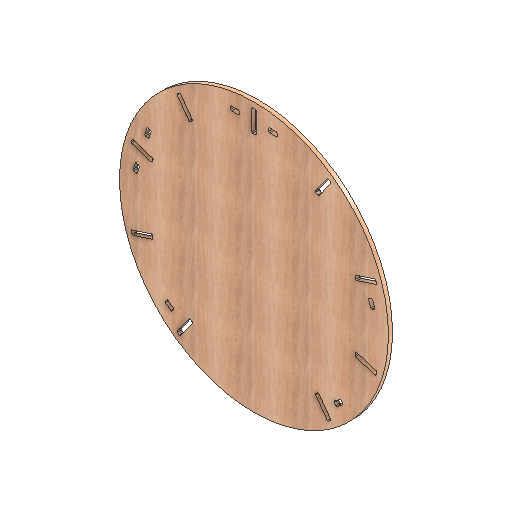
# Autodesk Inventor part: Disk A
Saved by Autodesk Inventor 2021 (Build 250183000, 183)
## iProperties
Created: 2020-05-09
Part Number: Disk A
Material: Wood (Birch)
Document SubType Name: Modeling
Designer: Dan Wikman
Density: 0.55 g/cm^3
Appearance: Birch - Natural Polished
Mass: 10982.9 g
Surface Area: 23369.1 cm^2
Volume: 19968.9 cm^3
Autodesk Inventor part; units mm, degrees
ref_plane "YZ Plane" through (0, 0, 0) normal (1, 0, 0) x (0, 1, 0)
ref_plane "XZ Plane" through (0, 0, 0) normal (0, 1, 0) x (-1, 0, 0)
ref_plane "XY Plane" through (0, 0, 0) normal (0, 0, 1) x (1, 0, 0)
sketch "CONTOURS" plane through (0, 0, 0) normal (0, 0, 1) x (1, 0, 0)
  circle A0 centre (1825, 610) radius 600
  constraints: 1 centre point
sketch "HOLES" plane through (0, 0, 0) normal (0, 0, 1) x (1, 0, 0)
  line L0 (2278.5732, 452.6363) -> (2364.1682, 424.8247)
  arc A0 (2364.1682, 424.8247) -> (2369.2085, 427.3929) centre (2365.4043, 428.6289) ccw
  line L1 (2369.2085, 427.3929) -> (2372.6077, 437.8545)
  arc A1 (2372.6077, 437.8545) -> (2370.0396, 442.8948) centre (2368.8035, 439.0906) ccw
  line L2 (2370.0396, 442.8948) -> (2284.4445, 470.7063)
  arc A2 (2284.4445, 470.7063) -> (2279.4042, 468.1382) centre (2283.2084, 466.9021) ccw
  line L3 (2279.4042, 468.1382) -> (2276.005, 457.6765)
  arc A3 (2276.005, 457.6765) -> (2278.5732, 452.6363) centre (2279.8092, 456.4405) ccw
  line L4 (1550.5477, 1003.9136) -> (1497.647, 1076.7251)
  arc A4 (1497.647, 1076.7251) -> (1492.0598, 1077.61) centre (1494.411, 1074.3739) ccw
  line L5 (1492.0598, 1077.61) -> (1483.1606, 1071.1444)
  arc A5 (1483.1606, 1071.1444) -> (1482.2757, 1065.5572) centre (1485.5118, 1067.9083) ccw
  line L6 (1482.2757, 1065.5572) -> (1535.1764, 992.7456)
  arc A6 (1535.1764, 992.7456) -> (1540.7636, 991.8607) centre (1538.4124, 995.0968) ccw
  line L7 (1540.7636, 991.8607) -> (1549.6628, 998.3263)
  arc A7 (1549.6628, 998.3263) -> (1550.5477, 1003.9136) centre (1547.3116, 1001.5624) ccw
  line L8 (1429.4456, 241.6508) -> (1435.9113, 250.55)
  arc A8 (1441.4985, 251.4349) -> (1435.9113, 250.55) centre (1439.1473, 248.1989) ccw
  line L9 (1441.4985, 251.4349) -> (1465.769, 233.8014)
  arc A9 (1466.6539, 228.2142) -> (1465.769, 233.8014) centre (1463.4178, 230.5653) ccw
  line L10 (1466.6539, 228.2142) -> (1460.1883, 219.315)
  arc A10 (1454.6011, 218.4301) -> (1460.1883, 219.315) centre (1456.9522, 221.6661) ccw
  line L11 (1454.6011, 218.4301) -> (1430.3305, 236.0636)
  arc A11 (1429.4456, 241.6508) -> (1430.3305, 236.0636) centre (1432.6817, 239.2997) ccw
  line L12 (2114.8236, 992.7456) -> (2167.7243, 1065.5572)
  arc A12 (2167.7243, 1065.5572) -> (2166.8394, 1071.1444) centre (2164.4882, 1067.9083) ccw
  line L13 (2166.8394, 1071.1444) -> (2157.9402, 1077.61)
  arc A13 (2157.9402, 1077.61) -> (2152.353, 1076.7251) centre (2155.589, 1074.3739) ccw
  line L14 (2152.353, 1076.7251) -> (2099.4523, 1003.9136)
  arc A14 (2099.4523, 1003.9136) -> (2100.3372, 998.3263) centre (2102.6884, 1001.5624) ccw
  line L15 (2100.3372, 998.3263) -> (2109.2364, 991.8607)
  arc A15 (2109.2364, 991.8607) -> (2114.8236, 992.7456) centre (2111.5876, 995.0968) ccw
  line L16 (1928.5, 1140.5018) -> (1928.5, 1129.5018)
  arc A16 (1924.5, 1125.5018) -> (1928.5, 1129.5018) centre (1924.5, 1129.5018) ccw
  line L17 (1924.5, 1125.5018) -> (1894.5, 1125.5018)
  arc A17 (1890.5, 1129.5018) -> (1894.5, 1125.5018) centre (1894.5, 1129.5018) ccw
  line L18 (1890.5, 1129.5018) -> (1890.5, 1140.5018)
  arc A18 (1894.5, 1144.5018) -> (1890.5, 1140.5018) centre (1894.5, 1140.5018) ccw
  line L19 (1894.5, 1144.5018) -> (1924.5, 1144.5018)
  arc A19 (1928.5, 1140.5018) -> (1924.5, 1144.5018) centre (1924.5, 1140.5018) ccw
  line L20 (2361.5204, 675.4997) -> (2351.0588, 672.1005)
  arc A20 (2346.0185, 674.6687) -> (2351.0588, 672.1005) centre (2349.8227, 675.9048) ccw
  line L21 (2346.0185, 674.6687) -> (2336.748, 703.2004)
  arc A21 (2339.3162, 708.2407) -> (2336.748, 703.2004) centre (2340.5522, 704.4364) ccw
  line L22 (2339.3162, 708.2407) -> (2349.7778, 711.6399)
  arc A22 (2354.8181, 709.0717) -> (2349.7778, 711.6399) centre (2351.0138, 707.8356) ccw
  line L23 (2354.8181, 709.0717) -> (2364.0886, 680.54)
  arc A23 (2361.5204, 675.4997) -> (2364.0886, 680.54) centre (2360.2844, 679.3039) ccw
  line L24 (1352.4461, 872.3684) -> (1362.9077, 868.9692)
  arc A24 (1365.4759, 863.9289) -> (1362.9077, 868.9692) centre (1361.6716, 865.165) ccw
  line L25 (1365.4759, 863.9289) -> (1356.2054, 835.3972)
  arc A25 (1351.1651, 832.8291) -> (1356.2054, 835.3972) centre (1352.4011, 836.6333) ccw
  line L26 (1351.1651, 832.8291) -> (1340.7034, 836.2283)
  arc A26 (1338.1353, 841.2686) -> (1340.7034, 836.2283) centre (1341.9395, 840.0325) ccw
  line L27 (1338.1353, 841.2686) -> (1347.4058, 869.8003)
  arc A27 (1352.4461, 872.3684) -> (1347.4058, 869.8003) centre (1351.21, 868.5642) ccw
  line L28 (1365.5555, 470.7063) -> (1279.9604, 442.8948)
  arc A28 (1279.9604, 442.8948) -> (1277.3923, 437.8545) centre (1281.1965, 439.0906) ccw
  line L29 (1277.3923, 437.8545) -> (1280.7915, 427.3929)
  arc A29 (1280.7915, 427.3929) -> (1285.8317, 424.8247) centre (1284.5957, 428.629) ccw
  line L30 (1285.8317, 424.8247) -> (1371.4268, 452.6363)
  arc A30 (1371.4268, 452.6363) -> (1373.995, 457.6766) centre (1370.1908, 456.4405) ccw
  line L31 (1373.995, 457.6766) -> (1370.5958, 468.1382)
  arc A31 (1370.5958, 468.1382) -> (1365.5555, 470.7063) centre (1366.7916, 466.9021) ccw
  line L32 (1549.6628, 221.6737) -> (1540.7636, 228.1393)
  arc A32 (1540.7636, 228.1393) -> (1535.1764, 227.2544) centre (1538.4124, 224.9032) ccw
  line L33 (1535.1764, 227.2544) -> (1482.2757, 154.4428)
  arc A33 (1482.2757, 154.4428) -> (1483.1606, 148.8556) centre (1485.5118, 152.0917) ccw
  line L34 (1483.1606, 148.8556) -> (1492.0598, 142.39)
  arc A34 (1492.0598, 142.39) -> (1497.647, 143.2749) centre (1494.4109, 145.6261) ccw
  line L35 (1497.647, 143.2749) -> (1550.5477, 216.0864)
  line L36 (1550.5477, 216.0864) -> (1550.5991, 216.1589)
  line L37 (1550.5991, 216.1589) -> (1550.6493, 216.233)
  line L38 (2167.7243, 154.4428) -> (2114.8236, 227.2544)
  arc A35 (1815.5, 1090.0018) -> (1819.5, 1086.0018) centre (1819.5, 1090.0018) ccw
  line L39 (1819.5, 1086.0018) -> (1830.5, 1086.0018)
  arc A36 (1830.5, 1086.0018) -> (1834.5, 1090.0018) centre (1830.5, 1090.0018) ccw
  line L40 (1834.5, 1090.0018) -> (1834.5, 1180.0018)
  arc A37 (1834.5, 1180.0018) -> (1830.5, 1184.0018) centre (1830.5, 1180.0018) ccw
  line L41 (1830.5, 1184.0018) -> (1819.5, 1184.0018)
  arc A38 (1819.5, 1184.0018) -> (1815.5, 1180.0018) centre (1819.5, 1180.0018) ccw
  line L42 (1815.5, 1180.0018) -> (1815.5, 1090.0018)
  line L43 (1815.5, 1090.0018) -> (1815.501, 1089.913)
  line L44 (1815.501, 1089.913) -> (1815.504, 1089.8235)
  arc A39 (1365.5555, 749.2937) -> (1370.5958, 751.8618) centre (1366.7916, 753.0979) ccw
  line L45 (1370.5958, 751.8618) -> (1373.995, 762.3235)
  arc A40 (1373.995, 762.3235) -> (1371.4268, 767.3637) centre (1370.1908, 763.5595) ccw
  line L46 (1371.4268, 767.3637) -> (1285.8318, 795.1753)
  arc A41 (1285.8318, 795.1753) -> (1280.7915, 792.6071) centre (1284.5957, 791.371) ccw
  line L47 (1280.7915, 792.6071) -> (1277.3923, 782.1455)
  arc A42 (1277.3923, 782.1455) -> (1279.9604, 777.1052) centre (1281.1965, 780.9094) ccw
  line L48 (1279.9604, 777.1052) -> (1365.5555, 749.2937)
  line L49 (1365.5555, 749.2937) -> (1365.6403, 749.2672)
  line L50 (1365.6403, 749.2672) -> (1365.7263, 749.2423)
  arc A43 (2278.5732, 767.3637) -> (2276.005, 762.3234) centre (2279.8092, 763.5595) ccw
  line L51 (2276.005, 762.3234) -> (2279.4042, 751.8618)
  arc A44 (2279.4042, 751.8618) -> (2284.4445, 749.2937) centre (2283.2084, 753.0979) ccw
  line L52 (2284.4445, 749.2937) -> (2370.0396, 777.1052)
  arc A45 (2370.0396, 777.1052) -> (2372.6077, 782.1455) centre (2368.8035, 780.9094) ccw
  line L53 (2372.6077, 782.1455) -> (2369.2085, 792.6071)
  arc A46 (2369.2085, 792.6071) -> (2364.1682, 795.1753) centre (2365.4043, 791.371) ccw
  line L54 (2364.1682, 795.1753) -> (2278.5732, 767.3637)
  line L55 (2278.5732, 767.3637) -> (2278.489, 767.3354)
  line L56 (2278.489, 767.3354) -> (2278.4048, 767.3049)
  line L57 (1303.9531, 674.5846) -> (1303.9815, 674.6687)
  line L58 (1303.9815, 674.6687) -> (1313.252, 703.2004)
  arc A47 (1313.252, 703.2004) -> (1310.6838, 708.2407) centre (1309.4478, 704.4365) ccw
  line L59 (1310.6838, 708.2407) -> (1300.2222, 711.6399)
  arc A48 (1300.2222, 711.6399) -> (1295.1819, 709.0717) centre (1298.9861, 707.8356) ccw
  line L60 (1295.1819, 709.0717) -> (1285.9114, 680.54)
  arc A49 (1285.9114, 680.54) -> (1288.4796, 675.4997) centre (1289.7156, 679.3039) ccw
  line L61 (1288.4796, 675.4997) -> (1298.9412, 672.1005)
  arc A50 (1298.9412, 672.1005) -> (1303.9815, 674.6687) centre (1300.1773, 675.9048) ccw
  arc A51 (2114.8236, 227.2544) -> (2109.2364, 228.1393) centre (2111.5876, 224.9032) ccw
  line L62 (2109.2364, 228.1393) -> (2100.3372, 221.6737)
  arc A52 (2100.3372, 221.6737) -> (2099.4523, 216.0864) centre (2102.6884, 218.4376) ccw
  line L63 (2099.4523, 216.0864) -> (2152.353, 143.2749)
  arc A53 (2152.353, 143.2749) -> (2157.9402, 142.39) centre (2155.589, 145.6261) ccw
  line L64 (2157.9402, 142.39) -> (2166.8394, 148.8556)
  arc A54 (2166.8394, 148.8556) -> (2167.7243, 154.4428) centre (2164.4882, 152.0917) ccw
  line L65 (2114.8236, 227.2544) -> (2114.7706, 227.3256)
  line L66 (2114.7706, 227.3256) -> (2114.7156, 227.3963)
  line L67 (1725.4112, 1125.5028) -> (1725.5, 1125.5018)
  line L68 (1725.5, 1125.5018) -> (1755.5, 1125.5018)
  arc A55 (1755.5, 1125.5018) -> (1759.5, 1129.5018) centre (1755.5, 1129.5018) ccw
  line L69 (1759.5, 1129.5018) -> (1759.5, 1140.5018)
  arc A56 (1759.5, 1140.5018) -> (1755.5, 1144.5018) centre (1755.5, 1140.5018) ccw
  line L70 (1755.5, 1144.5018) -> (1725.5, 1144.5018)
  arc A57 (1725.5, 1144.5018) -> (1721.5, 1140.5018) centre (1725.5, 1140.5018) ccw
  line L71 (1721.5, 1140.5018) -> (1721.5, 1129.5018)
  arc A58 (1721.5, 1129.5018) -> (1725.5, 1125.5018) centre (1725.5, 1129.5018) ccw
  line L72 (2208.5739, 251.4863) -> (2208.5015, 251.4349)
  line L73 (2208.5015, 251.4349) -> (2184.231, 233.8014)
  arc A59 (2184.231, 233.8014) -> (2183.3461, 228.2142) centre (2186.5822, 230.5653) ccw
  line L74 (2183.3461, 228.2142) -> (2189.8117, 219.315)
  arc A60 (2189.8117, 219.315) -> (2195.3989, 218.4301) centre (2193.0478, 221.6661) ccw
  line L75 (2195.3989, 218.4301) -> (2219.6694, 236.0636)
  arc A61 (2219.6694, 236.0636) -> (2220.5544, 241.6508) centre (2217.3183, 239.2997) ccw
  line L76 (2220.5544, 241.6508) -> (2214.0887, 250.55)
  arc A62 (2214.0887, 250.55) -> (2208.5015, 251.4349) centre (2210.8527, 248.1989) ccw
  line L77 (2284.4976, 864.0137) -> (2284.5241, 863.9289)
  line L78 (2284.5241, 863.9289) -> (2293.7946, 835.3972)
  arc A63 (2293.7946, 835.3972) -> (2298.8349, 832.8291) centre (2297.5989, 836.6333) ccw
  line L79 (2298.8349, 832.8291) -> (2309.2966, 836.2283)
  arc A64 (2309.2966, 836.2283) -> (2311.8647, 841.2686) centre (2308.0605, 840.0325) ccw
  line L80 (2311.8647, 841.2686) -> (2302.5942, 869.8003)
  arc A65 (2302.5942, 869.8003) -> (2297.5539, 872.3684) centre (2298.79, 868.5642) ccw
  line L81 (2297.5539, 872.3684) -> (2287.0923, 868.9692)
  arc A66 (2287.0923, 868.9692) -> (2284.5241, 863.9289) centre (2288.3284, 865.165) ccw
  arc A67 (1550.5477, 216.0864) -> (1549.6628, 221.6737) centre (1547.3116, 218.4376) ccw
  constraints: 164 end point, 150 point on circle, 68 centre point
sketch "LETTERS" plane through (0, 0, 0) normal (0, 0, 1) x (1, 0, 0)
  line L0 (1815.8805, 602.0819) -> (1824.962, 621.8307)
  line L1 (1824.962, 621.8307) -> (1834.2694, 602.0819)
  line L2 (1830.4476, 609.8529) -> (1819.5524, 609.8542)
  constraints: 6 end point
extrude "Extrusion1" add sketch "CONTOURS" along normal blind 18
extrude "Extrusion3" cut sketch "HOLES" along normal blind 18 contours A3 L3 A2 L2 A1 L1 A0 L0 | A7 L7 A6 L6 A5 L5 A4 L4 | L8 A8 L9 A9 L10 A10 L11 A11 | A15 L15 A14 L14 A13 L13 A12 L12 | L16 A16 L17 A17 L18 A18 L19 A19 | L20 A20 L21 A21 L22 A22 L23 A23 | L24 A24 L25 A25 L26 A26 L27 A27 | A31 L31 A30 L30 A29 L29 A28 L28 | A67 L37 L36 L35 A34 L34 A33 L33 A32 L32 | A54 L64 A53 L63 A52 L62 A51 L38 | L42 A38 L41 A37 L40 A36 L39 A35 | L48 A42 L47 A41 L46 A40 L45 A39 | L54 A46 L53 A45 L52 A44 L51 A43 | A50 L61 A49 L60 A48 L59 A47 L58 L57 | A58 L71 A57 L70 A56 L69 A55 L68 L67 | A62 L76 A61 L75 A60 L74 A59 L73 L72
body "Solid1"
